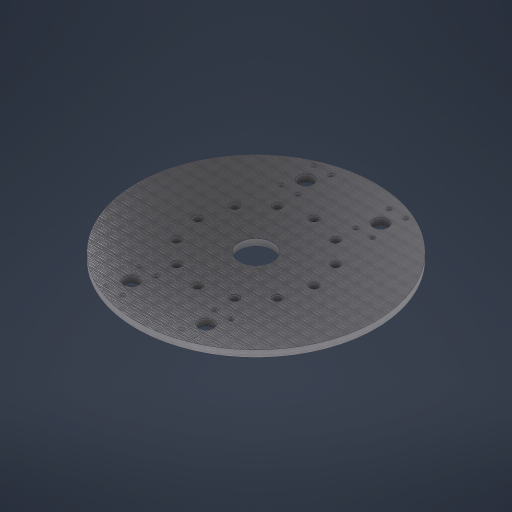
# Autodesk Inventor part: ArmBase
Saved by Autodesk Inventor 2024 (Build 280153000, 153)
## iProperties
Created: 2023-10-25
Part Number: ArmBase
Material: Generic
Document SubType Name: Modeling
Designer: avsar
Density: 1 g/cm^3
Appearance: Machined 03
Author: avsar
Autodesk Inventor part; units mm, degrees
ref_plane "YZ Plane" through (0, 0, 0) normal (1, 0, 0) x (0, 1, 0)
ref_plane "XZ Plane" through (0, 0, 0) normal (0, 1, 0) x (-1, 0, 0)
ref_plane "XY Plane" through (0, 0, 0) normal (0, 0, 1) x (1, 0, 0)
sketch "Sketch1" plane through (0, 0, 0) normal (0, 1, 0) x (-1, 0, 0)
  circle A0 centre (0, 0) radius 115
  circle A1 centre (0, 0) radius 16
  dimension "d0" = 230
  dimension "d1" = 32
  constraints: 2 centre point, 2 coincident
  measures "d0" diameter of A0
  measures "d1" diameter of A1
extrude "Extrusion1" add sketch "Sketch1" along normal blind 6.35
sketch "Sketch2" plane through (0, 6.35, 0) normal (0, 1, 0) x (1, 0, 0)
  circle A0 centre (0, 56) radius 4
  circle A1 centre (-28, 48.4974) radius 4
  circle A2 centre (-48.4974, 28) radius 4
  circle A3 centre (-56, 0) radius 4
  circle A4 centre (-48.4974, -28) radius 4
  circle A5 centre (-28, -48.4974) radius 4
  circle A6 centre (0, -56) radius 4
  circle A7 centre (28, -48.4974) radius 4
  circle A8 centre (48.4974, -28) radius 4
  circle A9 centre (56, 0) radius 4
  circle A10 centre (48.4974, 28) radius 4
  circle A11 centre (28, 48.4974) radius 4
  point P0 (0, 0)
  dimension "d4" = 8
  dimension "d5" = 56
  dimension "d8" = 360
  constraints: 12 centre point, 1 vertical alignment, 25 other
  measures "d4" diameter of A0
  measures "d5" distance of point (0, 0) A0.centre
extrude "Extrusion2" cut sketch "Sketch2" against normal through all
sketch "Sketch4" plane through (0, 6.35, 0) normal (0, 1, 0) x (1, 0, 0)
  circle A0 centre (-36, 84) radius 7
  circle A1 centre (-44, 100) radius 2
  line L0 (-36, 91) -> (-36, 77) construction
  line L1 (-43, 84) -> (-29, 84) construction
  circle A2 centre (-28, 100) radius 2
  circle A3 centre (-44, 68) radius 2
  circle A4 centre (-28, 68) radius 2
  circle A5 centre (0, 0) radius 16 construction
  line L2 (0, 16) -> (0, -16) construction
  line L3 (-16, 0) -> (16, 0) construction
  circle A6 centre (36, 84) radius 7
  circle A7 centre (44, 100) radius 2
  circle A8 centre (28, 100) radius 2
  circle A9 centre (44, 68) radius 2
  circle A10 centre (28, 68) radius 2
  circle A11 centre (-36, -84) radius 7
  circle A12 centre (-44, -100) radius 2
  circle A13 centre (-28, -100) radius 2
  circle A14 centre (-44, -68) radius 2
  circle A15 centre (-28, -68) radius 2
  circle A16 centre (36, -84) radius 7
  circle A17 centre (44, -100) radius 2
  circle A18 centre (28, -100) radius 2
  circle A19 centre (28, -68) radius 2
  circle A20 centre (44, -68) radius 2
  circle A21 centre (0, 0) radius 64 construction
  point P0 (-29, -84)
  dimension "d34" = 14
  dimension "d35" = 36
  dimension "d36" = 84
  dimension "d37" = 4
  dimension "d38" = 8
  dimension "d39" = 16
  dimension "d42" = 128
  constraints: 20 centre point, 19 symmetric about line, 8 end point, 8 point on circle, 4 midpoint, 3 coincident, 2 horizontal, 2 vertical, 1 horizontal alignment, 20 other
  measures "d34" diameter of A0
  measures "d35" horizontal distance of point (0, 0) A0.centre
  measures "d36" vertical distance of point (0, 0) A0.centre
  measures "d37" diameter of A1
  measures "d38" horizontal distance of A0.centre A1.centre
  measures "d39" vertical distance of A0.centre A1.centre
  measures "d42" diameter of A21
extrude "Extrusion4" cut sketch "Sketch4" against normal through all
body "Solid1"
